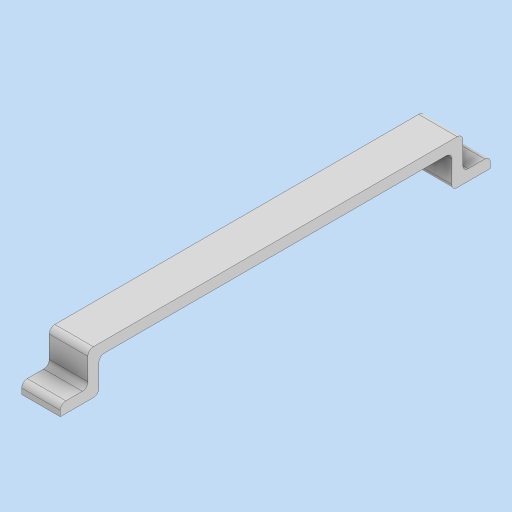
# Autodesk Inventor part: neotrellis_support
Saved by Autodesk Inventor 2024 (Build 280153000, 153)
## iProperties
Created: 2024-05-14
Part Number: neotrellis_support
Material: Generic
Document SubType Name: Modeling
Designer: fredyespana
Density: 1 g/cm^3
Appearance: Default
Author: fredyespana
Autodesk Inventor part; units mm, degrees
ref_plane "YZ Plane" through (0, 0, 0) normal (1, 0, 0) x (0, 1, 0)
ref_plane "XZ Plane" through (0, 0, 0) normal (0, 1, 0) x (-1, 0, 0)
ref_plane "XY Plane" through (0, 0, 0) normal (0, 0, 1) x (1, 0, 0)
sketch "Sketch1" plane through (0, 0, 0) normal (0, 1, 0) x (-1, 0, 0)
  line L0 (0, 39) -> (7, 39)
  line L1 (7, 39) -> (7, 32)
  line L2 (7, 32) -> (0, 32)
  line L3 (0, 32) -> (0, 39)
  line L4 (7, -32) -> (0, -32)
  line L5 (0, -32) -> (0, -39)
  line L6 (0, -39) -> (7, -39)
  line L7 (7, -39) -> (7, -32)
  line L8 (7, 32) -> (7, -32) construction
  point P0 (0, 0)
  point P1 (7, 0)
  dimension "d0" = 78
  dimension "d1" = 7
  constraints: 18 end point, 4 parallel, 3 equal length, 2 horizontal, 2 perpendicular, 1 horizontal alignment, 1 midpoint, 1 point on line, 1 vertical, 1 vertical alignment
  measures "d0" distance between parallel lines of L6 L0
  measures "d1" distance of L5.end L6.end
extrude "Extrusion1" add sketch "Sketch1" along normal blind 2
sketch "Sketch2" plane through (0, 2, 0) normal (0, 1, 0) x (1, 0, 0)
  line L0 (-7, -32) -> (-7, -39) projected
  line L1 (0, 32) -> (0, 39) projected
  line L2 (-7, -34) -> (0, -34)
  line L3 (0, -34) -> (0, 34)
  line L4 (0, 34) -> (-7, 34)
  line L5 (-7, 34) -> (-7, -34)
  line L6 (0, -32) -> (-7, -32) projected
  line L7 (-7, 32) -> (0, 32) projected
  point P0 (0, 0)
  dimension "d4" = 2
  dimension "d5" = 2
  constraints: 8 end point, 2 parallel, 2 point on line, 1 horizontal, 1 perpendicular
  measures "d4" distance between parallel lines of L2 L6
  measures "d5" distance between parallel lines of L4 L7
extrude "Extrusion2" add sketch "Sketch2" along normal blind 4 contours L6 L3 L2 L0 | L5 L4 L1 L7
sketch "Sketch3" plane through (0, 6, 0) normal (0, 1, 0) x (1, 0, 0)
  line L0 (-7, -34) -> (0, -34) projected
  line L1 (0, 34) -> (-7, 34) projected
  line L2 (0, -34) -> (-7, -34)
  line L3 (-7, -34) -> (-7, 34)
  line L4 (-7, 34) -> (0, 34)
  line L5 (0, 34) -> (0, -34)
  point P0 (0, 0)
  constraints: 8 end point, 2 parallel, 1 horizontal, 1 perpendicular
extrude "Extrusion3" add sketch "Sketch3" along normal blind 2
fillet "Fillet3" radius 1 9 edges at (-3.5, 2, 34) (-3.5, 2, 39) (-3.5, 2, -34) (-3.5, 0, 32) (-3.5, 0, -32) (-3.5, 6, -32) (-3.5, 6, 32) (-3.5, 8, -34) (-3.5, 8, 34)
fillet "Fillet4" radius 1 1 edges at (-3.5, 2, -39)
body "Solid1"
